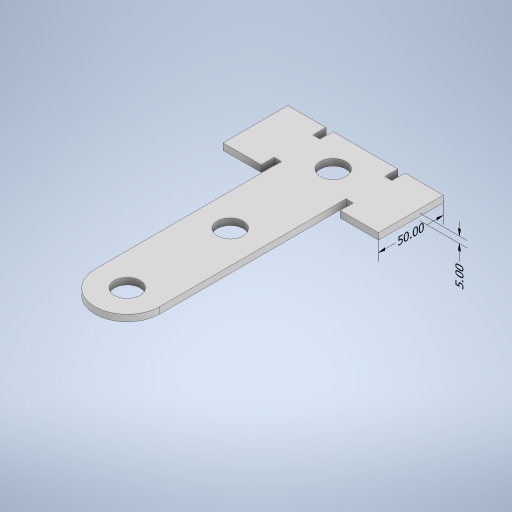
# Autodesk Inventor part: ギアプレート
Saved by Autodesk Inventor 2024.1 (Build 281209000, 209)
## iProperties
Created: 2024-04-01
Part Number: ギアプレート
Material: 一般
Document SubType Name: Modeling
Designer: hibik
Density: 1 g/cm^3
Appearance: 既定
Author: hibik
Autodesk Inventor part; units mm, degrees
ref_plane "YZ Plane" through (0, 0, 0) normal (1, 0, 0) x (0, 1, 0)
ref_plane "XZ Plane" through (0, 0, 0) normal (0, 1, 0) x (-1, 0, 0)
ref_plane "XY Plane" through (0, 0, 0) normal (0, 0, 1) x (1, 0, 0)
sketch "スケッチ1" plane through (0, 0, 0) normal (0, 1, 0) x (-1, 0, 0)
  line L0 (25, 0) -> (-25, 0)
  line L1 (-25, 0) -> (-25, -159)
  line L2 (-25, -159) -> (25, -159)
  line L3 (25, -159) -> (25, 0)
  circle A0 centre (0, 0) radius 25
  circle A1 centre (0, 0) radius 57 construction
  circle A2 centre (0, -79.5) radius 22.5 construction
  circle A3 centre (0, 0) radius 75 construction
  circle A4 centre (0, -79.5) radius 10
  circle A5 centre (0, 0) radius 10
  circle A6 centre (0, -159) radius 10
  circle A7 centre (0, -159) radius 57 construction
  circle A8 centre (0, -159) radius 25
  dimension "d0" = 114
  dimension "d1" = 45
  dimension "d2" = 150
  dimension "d3" = 20
  dimension "d4" = 20
  dimension "d5" = 50
  dimension "d8" = 20
  constraints: 8 centre point, 8 coincident, 8 end point, 3 tangent, 2 midpoint, 2 parallel, 2 vertical alignment, 1 equal radius, 1 horizontal, 1 perpendicular, 3 other
  measures "d0" diameter of A1
  measures "d1" diameter of A2
  measures "d2" diameter of A3
  measures "d3" diameter of A4
  measures "d4" diameter of A5
  measures "d5" distance of L1.end L2.end
  measures "d8" diameter of A6
extrude "押し出し1" add sketch "スケッチ1" along normal blind 5 contours A0 L0 A5 | L0 A5 A0 | L3 A8 L1 A0 | A8 L2 A6 | L2 A6 A8
sketch "スケッチ2" plane through (0, 0, 0) normal (0, -1, 0) x (1, 0, 0)
  line L0 (60, -134) -> (-60, -134)
  line L1 (-60, -134) -> (-60, -184)
  line L2 (-60, -184) -> (60, -184)
  line L3 (60, -184) -> (60, -134)
  line L4 (25, 0) -> (25, -159) projected
  arc A0 (25, 0) -> (-25, 0) centre (0, 0) ccw projected
  line L5 (-25, -159) -> (-25, 0) projected
  arc A1 (-25, -159) -> (25, -159) centre (0, -159) ccw projected
  circle A2 centre (0, 0) radius 10 projected
  circle A3 centre (0, -79.5) radius 10 projected
  circle A4 centre (0, -159) radius 10 projected
  arc A5 (-25, -159) -> (25, -159) centre (0, -159) ccw projected
  point P0 (0, -184)
  point P1 (25, -134)
  point P2 (0, -184)
  point P3 (-25, -134)
  dimension "d9" = 120
  dimension "d10" = 50
  constraints: 8 end point, 2 parallel, 1 horizontal, 1 midpoint, 1 perpendicular, 1 tangent, 1 vertical alignment
  measures "d9" distance of L1.end L2.end
  measures "d10" distance of L2.end L0.start
extrude "押し出し2" add sketch "スケッチ2" against normal up to surface (5 mm away) contours L3 L2 A1 L4 L0 | L5 A1 L2 L1 L0
sketch "スケッチ3" plane through (0, 5, 0) normal (0, 1, 0) x (1, 0, 0)
  line L0 (-60, 184) -> (60, 184) projected
  line L1 (-25, 134) -> (25, 134)
  line L2 (25, 134) -> (25, 184)
  line L3 (25, 184) -> (-25, 184)
  line L4 (-25, 184) -> (-25, 134)
  line L5 (-25, 184) -> (-30.5, 184)
  line L6 (-30.5, 184) -> (-30.5, 174)
  line L7 (-30.5, 174) -> (-25, 174)
  line L8 (-25, 174) -> (-25, 184)
  line L9 (25, 184) -> (30.5, 184)
  line L10 (30.5, 184) -> (30.5, 174)
  line L11 (30.5, 174) -> (25, 174)
  line L12 (25, 174) -> (25, 184)
  line L13 (-25, 134) -> (-60, 134) projected
  line L14 (-25, 134) -> (-30.5, 134)
  line L15 (-30.5, 134) -> (-30.5, 144)
  line L16 (-30.5, 144) -> (-25, 144)
  line L17 (-25, 144) -> (-25, 134)
  line L18 (25, 134) -> (30.5, 134)
  line L19 (30.5, 134) -> (30.5, 144)
  line L20 (30.5, 144) -> (25, 144)
  line L21 (25, 144) -> (25, 134)
  point P0 (0, 0)
  point P1 (25, 174)
  point P2 (-25, 144)
  point P3 (-25, 174)
  point P4 (-25, 184)
  dimension "d13" = 5.5
  dimension "d14" = 5.5
  dimension "d15" = 10
  constraints: 40 end point, 10 parallel, 5 horizontal, 5 perpendicular, 4 collinear, 3 point on line
  measures "d13" distance between parallel lines of L4 L6
  measures "d14" distance between parallel lines of L10 L12
  measures "d15" distance of L5.end L6.end
extrude "押し出し3" cut sketch "スケッチ3" against normal through all contours L0 L4 L7 L6 | L0 L10 L11 L2 | L4 L13 L15 L16 | L20 L19 L18 L2
equation "\"d14\" = d13"
